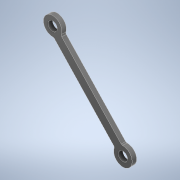
# Autodesk Inventor part: Pieza8
Saved by Autodesk Inventor 2022 (Build 260153000, 153)
## iProperties
Created: 2022-11-04
Part Number: Pieza8
Material: Resina acetálica, negra
Document SubType Name: Modeling
Designer: Mauricio Guerrero
Density: 1.425 g/cm^3
Appearance: Suave - Negro
Author: Mauricio Guerrero
## iProperties of the stored document Pieza8_3DPrint.ipt
Created: 2022-11-06
Part Number: Pieza8_3DPrint
Material: Genérico
Document SubType Name: Modeling
Designer: Mauricio Guerrero
Density: 1 g/cm^3
Appearance: Valor por defecto
Author: Mauricio Guerrero
Autodesk Inventor part; units mm, degrees
ref_plane "YZ Plane" through (0, 0, 0) normal (1, 0, 0) x (0, 1, 0)
ref_plane "XZ Plane" through (0, 0, 0) normal (0, 1, 0) x (-1, 0, 0)
ref_plane "XY Plane" through (0, 0, 0) normal (0, 0, 1) x (1, 0, 0)
sketch "Boceto1" plane through (0, 0, 0) normal (0, 0, 1) x (1, 0, 0)
  circle A0 centre (684.3626, 308.7393) radius 1.25
  arc A1 (686.7332, 307.9454) -> (684.4469, 306.2407) centre (684.3626, 308.7393) ccw
  circle A2 centre (703.3626, 287.7393) radius 1.25
  arc A3 (700.9878, 288.5205) -> (703.2626, 290.2373) centre (703.3626, 287.7393) ccw
  line L0 (684.3626, 308.7393) -> (703.3626, 287.7393) construction
  line L1 (689.4053, 303.1658) -> (691.9544, 305.4721) construction
  line L2 (686.8431, 307.4441) -> (702.8784, 290.3944)
  line L3 (684.828, 306.0836) -> (700.877, 289.0192)
  arc A4 (702.8784, 290.3944) -> (703.2626, 290.2373) centre (703.2426, 290.7369) ccw
  arc A5 (700.9878, 288.5205) -> (700.877, 289.0192) centre (700.5128, 288.6767) ccw
  arc A6 (686.7332, 307.9454) -> (686.8431, 307.4441) centre (687.2073, 307.7866) ccw
  arc A7 (684.828, 306.0836) -> (684.4469, 306.2407) centre (684.4637, 305.741) ccw
  point P0 (0, 0)
  point P1 (685.216, 309.1769)
  point P2 (703.1674, 288.8662)
  point P3 (683.8421, 307.9339)
  point P4 (702.2609, 288.0459)
  point P5 (686.6251, 307.6758)
  point P6 (684.6643, 306.2576)
  point P7 (701.0936, 288.7889)
  point P8 (703.0435, 290.2189)
  dimension "d7" = 2.5
  dimension "d8" = 5
  dimension "d10" = 5
  dimension "d11" = 19
  dimension "d12" = 21
  dimension "d14" = 2.4
  dimension "d15" = 0.5
  constraints: 16 point on circle, 8 centre point, 8 end point, 8 tangent, 5 point on line, 3 equal radius, 2 coincident, 2 symmetric about line, 1 perpendicular
  measures "d7" diameter of A0
  measures "d8" diameter of A1
  measures "d10" diameter of A3
  measures "d11" horizontal distance of A2.centre A0.centre
  measures "d12" vertical distance of A2.centre A0.centre
  measures "d14" distance between parallel lines of L2 L3
  measures "d15" radius of A4
extrude "Extrusión1" add sketch "Boceto1" along normal blind 1.2
